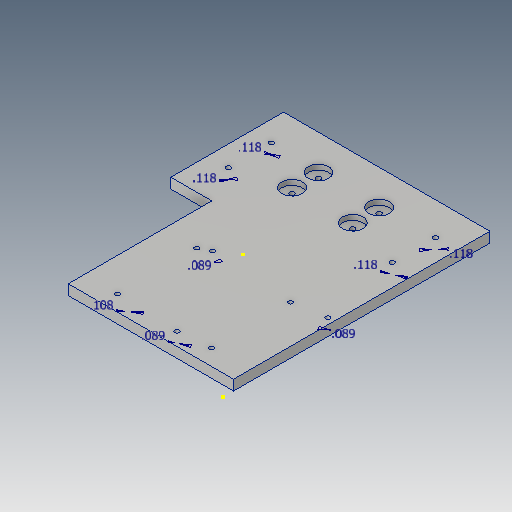
# Autodesk Inventor part: DPLX_P014_Lab_Baseplate_Small_PV
Saved by Autodesk Inventor 2018 (Build 220112000, 112)
## iProperties
Created: 2018-06-12
Part Number: DPLX_P014_Lab_Baseplate_Small_PV
Material: Aluminum 6061
Document SubType Name: Modeling
Designer: DPLXuser
Density: 2.7 g/cm^3
Appearance: Aluminum - Flat
Author: DPLXuser
Autodesk Inventor part; units mm, degrees
ref_plane "YZ Plane" through (0, 0, 0) normal (1, 0, 0) x (0, 1, 0)
ref_plane "XZ Plane" through (0, 0, 0) normal (0, 1, 0) x (-1, 0, 0)
ref_plane "XY Plane" through (0, 0, 0) normal (0, 0, 1) x (1, 0, 0)
sketch "Sketch1" plane through (0, 0, 0) normal (0, 1, 0) x (-1, 0, 0)
  line L0 (-63.881, 88.9) -> (63.881, 88.9)
  line L1 (63.881, 88.9) -> (63.881, -88.9)
  line L2 (63.881, -88.9) -> (-63.881, -88.9)
  line L3 (-63.881, -88.9) -> (-63.881, 88.9)
  line L4 (-63.881, 88.9) -> (63.881, -88.9) construction
  line L5 (63.881, 88.9) -> (-63.881, -88.9) construction
  point P0 (0, 0)
  dimension "d0" = 127.762
  dimension "d1" = 177.8
  constraints: 12 end point, 2 midpoint, 2 parallel, 1 horizontal, 1 perpendicular
  measures "d0" distance of L1.end L2.end
  measures "d1" distance of L0.end L1.end
extrude "Extrusion1" add sketch "Sketch1" along normal blind 6.35
sketch "Sketch4" plane through (0, 0, 0) normal (0, -1, 0) x (1, 0, 0)
  line L0 (63.881, 88.9) -> (-63.881, 88.9) projected
  line L1 (-63.881, 88.9) -> (-63.881, -88.9) projected
  line L2 (63.881, 88.9) -> (-63.881, 88.9)
  line L3 (-63.881, 88.9) -> (-63.881, 76.2)
  line L4 (-63.881, 76.2) -> (63.881, 76.2)
  line L5 (63.881, 76.2) -> (63.881, 88.9)
  point P0 (0, 0)
  point P1 (-59.9113, 88.9)
  point P2 (-63.881, 84.7576)
  dimension "d9" = 12.7
  constraints: 8 end point, 2 parallel, 1 horizontal, 1 perpendicular, 1 point on line
  measures "d9" distance of L3.end L0.end
extrude "Extrusion4" cut sketch "Sketch4" against normal blind 6.35
sketch "Sketch6" plane through (0, 0, 0) normal (0, -1, 0) x (1, 0, 0)
  circle A0 centre (-11.3792, 59.9948) radius 1.3716
  circle A1 centre (20.701, 61.722) radius 1.1303
  circle A2 centre (-11.303, 7.62) radius 1.1303
  circle A3 centre (60.071, 7.62) radius 1.1303
  circle A4 centre (-51.181, -41.91) radius 1.4986
  circle A5 centre (50.419, -41.91) radius 1.4986
  circle A6 centre (50.419, -68.58) radius 1.4986
  circle A7 centre (-51.181, -68.58) radius 1.4986
  point P0 (0, 0)
  point P1 (63.881, 76.2)
  dimension "d24" = 2.7432
  dimension "d26" = 2.2606
  dimension "d33" = 2.2606
  dimension "d34" = 2.2606
  dimension "d48" = 2.9972
  dimension "d49" = 2.9972
  dimension "d63" = 2.9972
  dimension "d64" = 2.9972
  constraints: 8 centre point
  measures "d24" diameter of A0
  measures "d26" diameter of A1
  measures "d33" diameter of A2
  measures "d34" diameter of A3
  measures "d48" diameter of A4
  measures "d49" diameter of A5
  measures "d63" diameter of A6
  measures "d64" diameter of A7
sketch "Sketch7" plane through (0, 6.35, 0) normal (0, 1, 0) x (1, 0, 0)
  line L0 (-63.881, -76.2) -> (63.881, -76.2) projected
  line L1 (-63.881, -76.2) -> (-63.881, 88.9) projected
  line L2 (63.881, -76.2) -> (-63.881, -76.2)
  line L3 (-63.881, -76.2) -> (-63.881, -69.85)
  line L4 (-63.881, -69.85) -> (63.881, -69.85)
  line L5 (63.881, -69.85) -> (63.881, -76.2)
  point P0 (0, 0)
  dimension "d204" = 6.35
  constraints: 8 end point, 2 parallel, 1 horizontal, 1 perpendicular, 1 point on line
  measures "d204" distance of L2.end L3.end
extrude "Extrusion7" cut sketch "Sketch7" against normal blind 25.4
sketch "Sketch8" plane through (0, 0, 0) normal (0, -1, 0) x (1, 0, 0)
  circle A0 centre (-20.701, -67.31) radius 1.4986
  circle A1 centre (-20.701, -50.9524) radius 1.4986
  circle A2 centre (16.891, -50.9524) radius 1.4986
  circle A3 centre (16.891, -67.31) radius 1.4986
  point P0 (0, 0)
  point P1 (-63.881, -88.9)
  dimension "d213" = 2.9972
  dimension "d216" = 2.9972
  dimension "d217" = 2.9972
  dimension "d218" = 2.9972
  constraints: 4 centre point
  measures "d213" diameter of A0
  measures "d216" diameter of A1
  measures "d217" diameter of A2
  measures "d218" diameter of A3
extrude "Extrusion8" cut sketch "Sketch8" against normal blind 25.4
sketch "Sketch9" plane through (0, 6.35, 0) normal (0, 1, 0) x (1, 0, 0)
  point P0 (0, 0)
sketch "Sketch10" plane through (0, 6.35, 0) normal (0, 1, 0) x (1, 0, 0)
  circle A0 centre (-20.701, 67.31) radius 1.4986 projected
  circle A1 centre (-20.701, 67.31) radius 6.35
  circle A2 centre (16.891, 67.31) radius 1.4986 projected
  circle A3 centre (16.891, 67.31) radius 6.35
  circle A4 centre (16.891, 50.9524) radius 1.4986 projected
  circle A5 centre (16.891, 50.9524) radius 6.35
  circle A6 centre (-20.701, 50.9524) radius 1.4986 projected
  circle A7 centre (-20.701, 50.9524) radius 6.35
  point P0 (0, 0)
  dimension "d221" = 12.7
  dimension "d222" = 12.7
  dimension "d223" = 12.7
  dimension "d224" = 12.7
  constraints: 4 centre point, 4 coincident
  measures "d221" diameter of A1
  measures "d222" diameter of A3
  measures "d223" diameter of A5
  measures "d224" diameter of A7
extrude "Extrusion9" cut sketch "Sketch10" against normal blind 3.175
extrude "Extrusion14" cut sketch "Sketch6" against normal blind 6.35 contours A4 | A5 | A6 | A7
sketch "Sketch13" plane through (0, 0, 0) normal (0, -1, 0) x (1, 0, 0)
  circle A0 centre (-51.181, -41.91) radius 1.4986 projected
  circle A1 centre (-51.181, -41.91) radius 6.35
  circle A2 centre (-51.181, -68.58) radius 1.4986 projected
  circle A3 centre (-51.181, -68.58) radius 6.35
  circle A4 centre (50.419, -68.58) radius 1.4986 projected
  circle A5 centre (50.419, -68.58) radius 6.35
  circle A6 centre (50.419, -41.91) radius 1.4986 projected
  circle A7 centre (50.419, -41.91) radius 6.35
  point P0 (0, 0)
  dimension "d247" = 12.7
  dimension "d248" = 12.7
  dimension "d249" = 12.7
  dimension "d250" = 12.7
  constraints: 4 centre point, 4 coincident
  measures "d247" diameter of A1
  measures "d248" diameter of A3
  measures "d249" diameter of A5
  measures "d250" diameter of A7
extrude "Extrusion15" cut sketch "Sketch13" against normal blind 3.175
sketch "Sketch14" plane through (0, 0, 0) normal (0, -1, 0) x (1, 0, 0)
  line L0 (-63.881, -88.9) -> (-63.881, 69.85) projected
  line L1 (-63.881, 69.85) -> (-38.481, 69.85)
  line L2 (-38.481, 69.85) -> (-38.481, -19.05)
  line L3 (-38.481, -19.05) -> (-63.881, -19.05)
  line L4 (-63.881, -19.05) -> (-63.881, 69.85)
  point P0 (0, 0)
  dimension "d253" = 25.4
  dimension "d254" = 88.9
  constraints: 8 end point, 2 parallel, 1 horizontal, 1 perpendicular
  measures "d253" distance of L2.end L3.end
  measures "d254" distance of L1.end L2.end
extrude "Extrusion16" cut sketch "Sketch14" against normal blind 6.35
sketch "Sketch15" plane through (0, 0, 0) normal (0, -1, 0) x (1, 0, 0)
  circle A0 centre (-11.3792, 59.9948) radius 1.3716 projected
  circle A1 centre (40.259, 59.9948) radius 1.3716
  circle A2 centre (-17.7292, 59.9948) radius 1.3716
  circle A3 centre (-17.7292, 10.9982) radius 1.3716
  circle A4 centre (40.259, 10.9982) radius 1.3716
  point P0 (0, 0)
  dimension "d262" = 2.7432
  dimension "d263" = 2.7432
  dimension "d264" = 2.7432
  dimension "d265" = 2.7432
  constraints: 4 centre point
  measures "d262" diameter of A1
  measures "d263" diameter of A2
  measures "d264" diameter of A3
  measures "d265" diameter of A4
extrude "Extrusion18" cut sketch "Sketch15" against normal blind 25.4 contours A1 | A2 | A3 | A4
hole "Hole17" at (20.701, 0, 61.722) at (60.071, 0, 7.62) at (-11.303, 0, 7.62) direction (0, 1, 0) diameter 2.7432 depth 6.35 countersink diameter 4.1148 countersink angle 82
body "Solid1"
